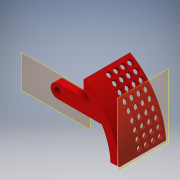
# Autodesk Inventor part: bumper_L
Saved by Autodesk Inventor 2016 (Build 200138000, 138)
## iProperties
Created: 2016-09-25
Part Number: bumper_L
Material: Generic
Document SubType Name: Modeling
Designer: benja
Density: 1 g/cm^3
Appearance: Red
Author: benja
Autodesk Inventor part; units mm, degrees
ref_plane "XZ Plane" through (0, 0, 0) normal (0, 1, 0) x (-1, 0, 0)
ref_plane "XY Plane" through (0, 0, 0) normal (0, 0, 1) x (1, 0, 0)
ref_plane "Work Plane1" through (0, 0, 0) normal (0, 0, 1) x (1, 0, 0)
sketch "Sketch1" plane through (0, 0, 0) normal (0, 0, 1) x (1, 0, 0)
  circle A0 centre (-7.3774, 2.1226) radius 1.75 projected
  circle A1 centre (2.6226, 2.1226) radius 1.75 projected
  circle A2 centre (2.6226, 2.1226) radius 1.75
  line L0 (22.0601, 5.8726) -> (2.6226, 5.8726)
  arc A3 (2.6226, 5.8726) -> (2.6226, -1.6274) centre (2.6226, 2.1226) ccw
  arc A4 (20.1226, -49.8774) -> (20.1226, 10.1226) centre (-2.3774, -19.8774) ccw projected
  arc A5 (38.0671, -17.7578) -> (17.6226, 15.3398) centre (-2.3774, -19.8774) ccw
  arc A6 (33.074, -18.0194) -> (17.6226, 9.4527) centre (-2.3774, -19.8774) ccw
  line L1 (17.6226, 9.4527) -> (17.6226, 15.3398)
  line L2 (15.6226, 7.1226) -> (15.6226, 15.4603) projected
  line L3 (33.074, -18.0194) -> (38.0671, -17.7578)
  line L4 (-2.3774, -19.8774) -> (39.7605, -19.8774)
  line L5 (2.6226, -1.6274) -> (28.0724, -1.6274)
  line L6 (17.6226, 5.8726) -> (17.6226, -1.6274)
  line L7 (20.6226, 5.8726) -> (20.6226, -1.6274)
  arc A7 (14.7573, 16.8194) -> (-19.512, 16.8194) centre (-2.3774, -19.8774) ccw projected
  arc A8 (8.6348, 5.3906) -> (9.6348, 5.1226) centre (9.6348, 7.1226) ccw projected
  line L8 (8.6348, 5.1226) -> (8.6348, 5.3906) projected
  line L9 (-13.3895, 5.1226) -> (8.6348, 5.1226) projected
  line L10 (-13.3895, 5.1226) -> (-13.3895, 5.3906) projected
  arc A9 (-14.3895, 5.1226) -> (-13.3895, 5.3906) centre (-14.3895, 7.1226) ccw projected
  line L11 (-19.3774, 5.1226) -> (-14.3895, 5.1226) projected
  line L12 (-19.3774, -0.8774) -> (-19.3774, 5.1226) projected
  line L13 (6.6226, -0.8774) -> (-19.3774, -0.8774) projected
  arc A10 (8.6226, -2.8774) -> (6.6226, -0.8774) centre (6.6226, -2.8774) ccw projected
  line L14 (8.6226, -9.8774) -> (8.6226, -2.8774) projected
  line L15 (14.6226, -9.8774) -> (8.6226, -9.8774) projected
  line L16 (14.6226, 5.1226) -> (14.6226, -9.8774) projected
  line L17 (9.6348, 5.1226) -> (14.6226, 5.1226) projected
  point P0 (0, 0)
  dimension "d0" = 3.5
  dimension "d1" = 2
  dimension "d2" = 2
  dimension "d5" = 3
  dimension "d6" = 2
  dimension "d8" = 3
  constraints: 14 end point, 8 point on circle, 4 centre point, 4 coincident, 4 point on line, 3 tangent, 2 horizontal, 2 perpendicular, 1 line through centre, 1 parallel, 1 vertical
  measures "d0" diameter of A2
  measures "d1" radial gap between concentric circles of A1 A3
  measures "d2" distance between parallel lines of L1 L2
  measures "d5" angle of L4 L3
  measures "d6" radial gap between concentric circles of A4 A6
  measures "d8" distance between parallel lines of L6 L7
extrude "Extrusion1" add sketch "Sketch1" along normal blind 4 contours A6 L5 L7 L0 | A6 L1 A5 L3 | L7 L5 L6 L0 | L6 L5 L16 L17 A8 L8 L9 A3 L0 | L9 L8 A8 L17 L16 L5 A10 L13 A3 | L13 A10 L5 A3
sketch "Sketch2" plane through (0, 0, 0) normal (0, 0, -1) x (-1, 0, 0)
  circle A0 centre (-2.6226, 2.1226) radius 1.75 projected
  line L0 (-22.0601, 5.8726) -> (-2.6226, 5.8726) projected
  arc A1 (-17.6226, 9.4527) -> (-22.0601, 5.8726) centre (2.3774, -19.8774) ccw projected
  line L1 (-17.6226, 15.3398) -> (-17.6226, 9.4527) projected
  arc A2 (-17.6226, 15.3398) -> (-38.0671, -17.7578) centre (2.3774, -19.8774) ccw projected
  line L2 (-33.074, -18.0194) -> (-38.0671, -17.7578) projected
  arc A3 (-28.0724, -1.6274) -> (-33.074, -18.0194) centre (2.3774, -19.8774) ccw projected
  line L3 (-2.6226, -1.6274) -> (-28.0724, -1.6274) projected
  arc A4 (-2.6226, -1.6274) -> (-2.6226, 5.8726) centre (-2.6226, 2.1226) ccw projected
  line L4 (-15.6226, -10.8774) -> (-15.6226, 6.1226) projected
  line L5 (-2.6226, -1.6274) -> (-28.0724, -1.6274) projected
  line L6 (-18.6226, -1.6274) -> (-18.6226, 5.8726)
  line L7 (-22.0601, 5.8726) -> (-2.6226, 5.8726) projected
  point P0 (0, 0)
  dimension "d11" = 3
  constraints: 2 end point, 2 point on line, 1 perpendicular
  measures "d11" distance between parallel lines of L4 L6
extrude "Extrusion2" add sketch "Sketch2" along normal blind 4.5 contours L0 L6 L3 A3 L2 A2 L1 A1
sketch "Sketch3" plane through (0, 0, -4.5) normal (0, 0, -1) x (-1, 0, 0)
  arc A0 (-17.6226, 9.4527) -> (-22.0601, 5.8726) centre (2.3774, -19.8774) ccw projected
  line L0 (-17.6226, 9.4527) -> (-17.6226, 15.3398) projected
  arc A1 (-17.6226, 15.3398) -> (-38.0671, -17.7578) centre (2.3774, -19.8774) ccw projected
  line L1 (-38.0671, -17.7578) -> (-33.074, -18.0194) projected
  arc A2 (-28.0724, -1.6274) -> (-33.074, -18.0194) centre (2.3774, -19.8774) ccw projected
  line L2 (-28.0724, -1.6274) -> (-18.6226, -1.6274) projected
  line L3 (-18.6226, -1.6274) -> (-18.6226, 5.8726) projected
  line L4 (-18.6226, 5.8726) -> (-22.0601, 5.8726) projected
  line L5 (-38.0671, -17.7578) -> (-33.074, -18.0194) projected
  arc A3 (-17.6226, 13.604) -> (-36.5692, -17.8363) centre (2.3774, -19.8774) ccw
  line L6 (-17.6226, 9.4527) -> (-17.6226, 15.3398) projected
  line L7 (-17.6226, 13.604) -> (-17.6226, 15.3398)
  line L8 (-36.5692, -17.8363) -> (-38.0671, -17.7578)
  point P0 (0, 0)
  dimension "d14" = 1.5
  constraints: 4 end point, 2 collinear, 2 point on circle, 1 centre point, 1 coincident, 1 point on line
  measures "d14" radial gap between concentric circles of A1 A3
extrude "Extrusion3" add sketch "Sketch3" along normal blind 18 contours A3 L1 A1 L0
ref_plane "Work Plane2" through (38.1226, -19.8774, 0) normal (1, 0, 0) x (0, 1, 0)
sketch "Sketch4" plane through (38.1226, -19.8774, 0) normal (1, 0, 0) x (0, 1, 0)
  circle A0 centre (5.1196, -7.6) radius 1.5
  line L0 (35.2172, -22.5) -> (35.2172, 4) projected
  line L1 (2.1196, 4) -> (35.2172, 4) projected
  line L2 (2.1196, -22.5) -> (2.1196, 4) projected
  line L3 (35.2172, -22.5) -> (2.1196, -22.5) projected
  line L4 (-30, -5) -> (30, -5) projected
  point P0 (19.8774, 0)
  dimension "d17" = 3
  dimension "d18" = 33.0976
  dimension "d21" = 1.5
  dimension "d27" = 17.5
  dimension "d28" = 1.1
  constraints: 1 centre point
  measures "d17" diameter of A0
  measures "d18" distance of L0.start L2.start
  measures "d21" distance edge to line of A0 L2
  measures "d27" distance between parallel lines of L3 L4
  measures "d28" distance edge to line of A0 L4
extrude "Extrusion4" cut sketch "Sketch4" against normal through all contours A0
pattern_linear "Rectangular Pattern1" count 4 spacing 4 along (0, 0, -1) of "Extrusion4"
pattern_circular "Circular Pattern1" count 9 over 48 about axis through (-2.3774, -19.8774, 0) along (0, 0, 1) of "Extrusion4", "Rectangular Pattern1"
body "Solid1"
